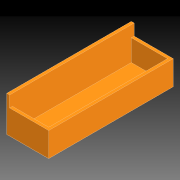
# Autodesk Inventor part: KB33-046-008-001 - Корпус
Saved by Autodesk Inventor 2020 (Build 240168000, 168)
## iProperties
Created: 2021-08-09
Part Number: KB33-046-008-001 - Корпус
Material: Типовые
Document SubType Name: Modeling
Designer: Петров Иван
Mass: 211.32 g
Surface Area: 876.68 cm^2
Volume: 211.32 cm^3
Density: 1 g/cm^3
Appearance: Оранжевый
Author: Петров Иван
Autodesk Inventor part; units mm, degrees
ref_plane "YZ Plane" through (0, 0, 0) normal (1, 0, 0) x (0, 1, 0)
ref_plane "XZ Plane" through (0, 0, 0) normal (0, 1, 0) x (-1, 0, 0)
ref_plane "XY Plane" through (0, 0, 0) normal (0, 0, 1) x (1, 0, 0)
sketch "Эскиз1" plane through (0, 0, 0) normal (0, 1, 0) x (-1, 0, 0)
  line L0 (-37, 110) -> (37, 110)
  line L1 (37, 110) -> (37, -110)
  line L2 (37, -110) -> (-37, -110)
  line L3 (-37, -110) -> (-37, 110)
  line L4 (-37, 110) -> (37, -110) construction
  line L5 (37, 110) -> (-37, -110) construction
  point P0 (0, 0)
  dimension "d0" = 74
  dimension "d1" = 220
  constraints: 12 end point, 2 midpoint, 2 parallel, 1 horizontal, 1 perpendicular
  measures "d0" distance of L1.end L2.end
  measures "d1" distance of L0.end L1.end
extrude "Выдавливание1" add sketch "Эскиз1" along normal blind 43
sketch "Эскиз3" plane through (0, 43, 0) normal (0, 1, 0) x (1, 0, 0)
  line L0 (-32, -105) -> (32, -105)
  line L1 (32, -105) -> (32, 105)
  line L2 (32, 105) -> (-32, 105)
  line L3 (-32, 105) -> (-32, -105)
  line L4 (-32, -105) -> (32, 105) construction
  line L5 (32, -105) -> (-32, 105) construction
  line L6 (37, 110) -> (-37, 110) projected
  line L7 (-37, 110) -> (-37, -110) projected
  point P0 (0, 0)
  dimension "d4" = 5
  dimension "d5" = 5
  constraints: 12 end point, 2 midpoint, 2 parallel, 1 horizontal, 1 perpendicular
  measures "d4" distance between parallel lines of L6 L2
  measures "d5" distance between parallel lines of L7 L3
extrude "Выдавливание2" cut sketch "Эскиз3" against normal blind 38
sketch "Эскиз4" plane through (0, 5, 0) normal (0, 1, 0) x (1, 0, 0)
  line L0 (32, 105) -> (32, -105) projected
  line L1 (32, 105) -> (0, 105)
  line L2 (0, 105) -> (0, 67.1211)
  line L3 (0, 67.1211) -> (32, 67.1211)
  line L4 (32, 67.1211) -> (32, 105)
  point P0 (0, 0)
  constraints: 8 end point, 2 parallel, 1 horizontal, 1 perpendicular
sketch "Эскиз5" plane through (0, 43, 0) normal (0, 1, 0) x (1, 0, 0)
  line L0 (-37, 110) -> (-37, -110) projected
  line L1 (-37, -110) -> (37, -110) projected
  line L2 (-37, 110) -> (-32, 110)
  line L3 (-32, 110) -> (-32, -110)
  line L4 (-32, -110) -> (-37, -110)
  line L5 (-37, -110) -> (-37, 110)
  line L6 (-32, -105) -> (-32, 105) projected
  point P0 (0, 0)
  point P1 (-32, 0)
  constraints: 8 end point, 2 midpoint, 2 parallel, 1 horizontal, 1 perpendicular, 1 point on line
extrude "Выдавливание3" add sketch "Эскиз5" along normal blind 20
